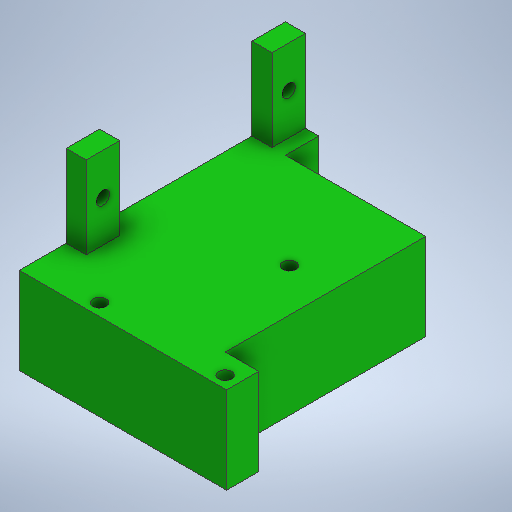
# Autodesk Inventor part: spojene 2
Saved by Autodesk Inventor 2026.1 (Build 301233020, 233B)
## iProperties
Created: 2025-07-05
Part Number: spojene 2
Material: Generic
Document SubType Name: Modeling
Designer: admin
Density: 1 g/cm^3
Appearance: Default
Author: admin
Autodesk Inventor part; units mm, degrees
ref_plane "YZ Plane" through (0, 0, 0) normal (1, 0, 0) x (0, 1, 0)
ref_plane "XZ Plane" through (0, 0, 0) normal (0, 1, 0) x (-1, 0, 0)
ref_plane "XY Plane" through (0, 0, 0) normal (0, 0, 1) x (1, 0, 0)
sketch "Sketch1" plane through (0, 0, 0) normal (0, 1, 0) x (-1, 0, 0)
  line L0 (9, -28.2161) -> (9, 11.5839)
  line L1 (9, 11.5839) -> (4, 11.5839)
  line L2 (4, 11.5839) -> (4, 11.5839)
  line L3 (4, 11.5839) -> (-22, 11.5839)
  line L4 (9, -28.2161) -> (4, -28.2161)
  line L5 (4, -28.2161) -> (4, -23.2161)
  line L6 (-22, 6.7839) -> (-22, 11.5839)
  line L7 (4, -23.2161) -> (-17, -23.2161)
  line L8 (-17, -23.2161) -> (-17, 6.7839)
  line L9 (-17, 6.7839) -> (-22, 6.7839)
  point P0 (0, 0)
  dimension "d28" = 0
  dimension "d30" = 5
  dimension "d69" = 5
  dimension "d98" = 5
  dimension "d101" = 21
  dimension "d102" = 30
  constraints: 20 end point, 4 perpendicular, 2 horizontal, 1 vertical
  measures "d28" distance of L1.end L2.end
  measures "d30" distance of L4.end L5.end
  measures "d69" distance between parallel lines of L2 L0
  measures "d98" distance of L0.start L4.end
  measures "d101" distance of L5.end L7.end
  measures "d102" distance of L7.end L8.end
extrude "Extrusion1" add sketch "Sketch1" along normal blind 13
sketch "Sketch7" plane through (0, 13, 0) normal (0, 1, 0) x (1, 0, 0)
  circle A0 centre (1.2, -9.7839) radius 1
  circle A1 centre (20, -9.7839) radius 1
  circle A2 centre (10.6, 9.2161) radius 1
  line L0 (22, 11.2161) -> (-4, 11.2161) projected
  line L1 (-9, 28.2161) -> (-9, -11.5839) projected
  line L2 (22, -11.5839) -> (22, 11.2161) projected
  point P0 (0, 0)
  point P1 (-4, 23.2161)
  point P2 (-9, 23.2161)
  point P3 (-9, -6.5839)
  dimension "d84" = 2
  dimension "d85" = 2
  dimension "d87" = 2
  dimension "d88" = 19
  dimension "d89" = 9.4
  dimension "d90" = 2
  dimension "d91" = 19
  dimension "d93" = 9.4
  dimension "d100" = 2
  constraints: 3 centre point
  measures "d84" diameter of A0
  measures "d85" diameter of A1
  measures "d87" diameter of A2
  measures "d88" vertical distance of A0.centre A2.centre
  measures "d89" horizontal distance of A0.centre A2.centre
  measures "d90" distance from line of L0 A2.centre
  measures "d91" vertical distance of A1.centre A2.centre
  measures "d93" horizontal distance of A2.centre A1.centre
  measures "d100" distance from line of L2 A1.centre
extrude "Extrusion8" cut sketch "Sketch7" against normal blind 15
sketch "Sketch8" plane through (0, 13, 0) normal (0, 1, 0) x (1, 0, 0)
  line L0 (-4, 28.2161) -> (-9, 28.2161) projected
  line L1 (-9, 28.2161) -> (-6, 28.2161)
  line L2 (-6, 28.2161) -> (-6, 23.2161)
  line L3 (-6, 23.2161) -> (-9, 23.2161)
  line L4 (-9, 23.2161) -> (-9, 28.2161)
  line L5 (-9, 28.2161) -> (-9, -11.5839) projected
  line L6 (-6, -4.5839) -> (-9, -4.5839)
  line L7 (-9, -4.5839) -> (-9, 0.4161)
  line L8 (-9, 0.4161) -> (-6, 0.4161)
  line L9 (-6, 0.4161) -> (-6, -4.5839)
  point P0 (0, 0)
  dimension "d103" = 3
  dimension "d104" = 5
  dimension "d105" = 5
  dimension "d106" = 3
  dimension "d107" = 22.8
  constraints: 16 end point, 4 parallel, 2 horizontal, 2 perpendicular, 1 point on line
  measures "d103" distance of L2.end L3.end
  measures "d104" distance of L1.end L2.end
  measures "d105" distance of L8.end L6.start
  measures "d106" distance of L7.end L8.end
  measures "d107" distance between parallel lines of L3 L8
extrude "Extrusion9" add sketch "Sketch8" along normal blind 12.3
sketch "Sketch9" plane through (-9, 0, -28.2161) normal (-1, 0, 0) x (0, 0, 1)
  circle A0 centre (30.3, 19.15) radius 1
  line L0 (32.8, 13) -> (32.8, 25.3) projected
  line L1 (32.8, 13) -> (39.8, 13) projected
  circle A1 centre (2.5, 19.15) radius 1
  line L2 (5, 13) -> (27.8, 13) projected
  line L3 (5, 13) -> (5, 25.3) projected
  point P0 (28.2161, 0)
  dimension "d110" = 2
  dimension "d111" = 2.5
  dimension "d112" = 6.15
  dimension "d113" = 2
  dimension "d114" = 6.15
  dimension "d115" = 2.5
  constraints: 2 centre point
  measures "d110" diameter of A0
  measures "d111" distance from line of L0 A0.centre
  measures "d112" distance from line of L1 A0.centre
  measures "d113" diameter of A1
  measures "d114" distance from line of L2 A1.centre
  measures "d115" distance from line of L3 A1.centre
extrude "Extrusion10" cut sketch "Sketch9" against normal blind 12.3
body "Solid1"
